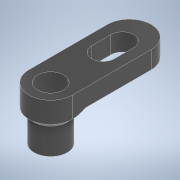
# Autodesk Inventor part: Servo steering actuator
Saved by Autodesk Inventor 2022.6 (Build 266554000, 554)
## iProperties
Created: 2024-11-03
Part Number: Servo steering actuator
Material: Generic
Document SubType Name: Modeling
Designer: Zhong
Density: 1 g/cm^3
Appearance: Dark Gray
Author: Zhong
Autodesk Inventor part; units mm, degrees
ref_plane "YZ Plane" through (0, 0, 0) normal (1, 0, 0) x (0, 1, 0)
ref_plane "XZ Plane" through (0, 0, 0) normal (0, 1, 0) x (-1, 0, 0)
ref_plane "XY Plane" through (0, 0, 0) normal (0, 0, 1) x (1, 0, 0)
sketch "Sketch1" plane through (0, 0, 0) normal (0, 1, 0) x (-1, 0, 0)
  circle A0 centre (0, 0) radius 1.4
  circle A1 centre (0, 0) radius 5
  circle A2 centre (0, -18) radius 5
  line L0 (5, 0) -> (5, -18)
  line L1 (-5, -18) -> (-5, 0)
  dimension "d0" = 2.8
  dimension "d1" = 10
  dimension "d3" = 18
  constraints: 4 end point, 4 point on circle, 4 tangent, 3 centre point, 2 coincident, 1 equal radius, 1 vertical alignment
  measures "d0" diameter of A0
  measures "d1" diameter of A1
  measures "d3" distance of point (0, 0) A2.centre
extrude "Extrusion1" add sketch "Sketch1" along normal blind 4
sketch "Sketch2" plane through (0, 4, 0) normal (0, 1, 0) x (1, 0, 0)
  line L0 (-5, 18) -> (-5, 0) projected
  arc A0 (-5, 0) -> (5, 0) centre (0, 0) ccw projected
  line L1 (5, 0) -> (5, 18) projected
  arc A1 (5, 18) -> (-5, 18) centre (0, 18) ccw projected
  circle A2 centre (0, 0) radius 1.4 projected
  line L2 (0, 16.4) -> (0, 12) construction
  line L3 (-2.6, 16.4) -> (-2.6, 12)
  line L4 (2.6, 12) -> (2.6, 16.4)
  arc A3 (2.6, 16.4) -> (-2.6, 16.4) centre (0, 16.4) ccw
  arc A4 (-2.6, 12) -> (2.6, 12) centre (0, 12) ccw
  point P0 (0, 14.2)
  dimension "d6" = 4.4
  dimension "d7" = 5.2
  dimension "d9" = 12
  constraints: 8 end point, 4 point on circle, 4 tangent, 2 centre point, 1 midpoint, 1 parallel, 1 vertical, 1 vertical alignment
  measures "d6" distance of L2.start L2.end
  measures "d7" diameter of A4
  measures "d9" distance of point (0, 0) L2.end
extrude "Extrusion2" cut sketch "Sketch2" against normal through all contours A3 L4 A4 L3
sketch "Sketch4" plane through (0, 0, 0) normal (0, -1, 0) x (1, 0, 0)
  line L0 (2.6, -12) -> (2.6, -16.4) projected
  arc A0 (-2.6, -16.4) -> (2.6, -16.4) centre (0, -16.4) ccw projected
  line L1 (-2.6, -16.4) -> (-2.6, -12) projected
  arc A1 (2.6, -12) -> (-2.6, -12) centre (0, -12) ccw projected
  line L2 (-5, -18) -> (-5, 0) projected
  arc A2 (-5, -18) -> (5, -18) centre (0, -18) ccw projected
  line L3 (5, 0) -> (5, -18) projected
  arc A3 (5, 0) -> (-5, 0) centre (0, 0) ccw projected
  circle A4 centre (0, 0) radius 1.4 projected
  arc A5 (5, 0) -> (-5, 0) centre (0, 0) ccw projected
  circle A6 centre (0, 0) radius 1.4 projected
  circle A7 centre (0, 0) radius 3.8
  circle A8 centre (0, 0) radius 1.4
  dimension "d39" = 7.6
  constraints: 2 centre point, 2 coincident, 1 concentric
  measures "d39" diameter of A7
extrude "Extrusion4" add sketch "Sketch4" along normal blind 8 contours A7
sketch "Sketch5" plane through (0, -8, 0) normal (0, -1, 0) x (1, 0, 0)
  circle A0 centre (0, 0) radius 1.4 projected
  circle A1 centre (0, 0) radius 2.5
  dimension "d17" = 5
  constraints: 1 centre point, 1 coincident
  measures "d17" diameter of A1
extrude "Extrusion5" cut sketch "Sketch5" against normal blind 5
sketch "Sketch6" plane through (0, 4, 0) normal (0, 1, 0) x (1, 0, 0)
  arc A0 (-5, 0) -> (5, 0) centre (0, 0) ccw projected
  line L0 (2.6, 16.4) -> (2.6, 12) projected
  arc A1 (-2.6, 12) -> (2.6, 12) centre (0, 12) ccw projected
  line L1 (-2.6, 12) -> (-2.6, 16.4) projected
  arc A2 (2.6, 16.4) -> (-2.6, 16.4) centre (0, 16.4) ccw projected
  line L2 (-5, 18) -> (-5, 0) projected
  arc A3 (-5, 0) -> (5, 0) centre (0, 0) ccw projected
  line L3 (5, 0) -> (5, 18) projected
  arc A4 (5, 18) -> (-5, 18) centre (0, 18) ccw projected
  circle A5 centre (0, 0) radius 1.4 projected
  circle A6 centre (0, 0) radius 1.4 projected
  circle A7 centre (0, 0) radius 3
  dimension "d20" = 6
  constraints: 1 centre point, 1 coincident
  measures "d20" diameter of A7
extrude "Extrusion6" cut sketch "Sketch6" against normal blind 5 contours A7
sketch "Sketch7" plane through (0, -8, 0) normal (0, -1, 0) x (1, 0, 0)
  circle A0 centre (0, 0) radius 2.5 projected
  circle A1 centre (0, 0) radius 2.9
  line L0 (1.9156, 2.1773) -> (1.9156, 1.7248)
  line L1 (1.9156, 1.7248) -> (2.3656, 1.6775)
  line L2 (1.4471, 2.1331) -> (1.8954, 2.1949)
  line L3 (1.3389, 2.5724) -> (1.4471, 2.1331)
  line L4 (0.8946, 2.4174) -> (1.315, 2.5847)
  line L5 (0.6843, 2.8181) -> (0.8946, 2.4174)
  line L6 (0.2901, 2.5613) -> (0.6583, 2.8243)
  line L7 (-0.01, 2.9) -> (0.2901, 2.5613)
  line L8 (-0.3313, 2.5563) -> (-0.0368, 2.8998)
  line L9 (-0.7037, 2.8133) -> (-0.3313, 2.5563)
  line L10 (-0.9334, 2.4027) -> (-0.7296, 2.8067)
  line L11 (-1.3565, 2.5632) -> (-0.9334, 2.4027)
  line L12 (-1.4813, 2.1095) -> (-1.3801, 2.5505)
  line L13 (-1.9305, 2.1641) -> (-1.4813, 2.1095)
  line L14 (-1.9431, 1.6937) -> (-1.9504, 2.1461)
  line L15 (-2.3923, 1.6392) -> (-1.9431, 1.6937)
  line L16 (-2.292, 1.1795) -> (-2.4073, 1.617)
  line L17 (-2.7151, 1.019) -> (-2.292, 1.1795)
  line L18 (-2.5077, 0.5967) -> (-2.7244, 0.9939)
  line L19 (-2.88, 0.3397) -> (-2.5077, 0.5967)
  line L20 (-2.5776, -0.0208) -> (-2.8831, 0.313)
  line L21 (-2.8776, -0.3594) -> (-2.5776, -0.0208)
  line L22 (-2.4977, -0.637) -> (-2.8742, -0.386)
  line L23 (-2.708, -1.0377) -> (-2.4977, -0.637)
  line L24 (-2.2727, -1.2163) -> (-2.6983, -1.0626)
  line L25 (-2.381, -1.6556) -> (-2.2727, -1.2163)
  line L26 (-1.9156, -1.7248) -> (-2.3656, -1.6775)
  line L27 (-1.9156, -2.1773) -> (-1.9156, -1.7248)
  line L28 (-1.4471, -2.1331) -> (-1.8954, -2.1949)
  line L29 (-1.3389, -2.5724) -> (-1.4471, -2.1331)
  line L30 (-0.8946, -2.4174) -> (-1.315, -2.5847)
  line L31 (-0.6843, -2.8181) -> (-0.8946, -2.4174)
  line L32 (-0.2901, -2.5613) -> (-0.6583, -2.8243)
  line L33 (0.01, -2.9) -> (-0.2901, -2.5613)
  line L34 (0.3313, -2.5563) -> (0.0368, -2.8998)
  line L35 (0.7037, -2.8133) -> (0.3313, -2.5563)
  line L36 (0.9334, -2.4027) -> (0.7296, -2.8067)
  line L37 (1.3565, -2.5632) -> (0.9334, -2.4027)
  line L38 (1.4813, -2.1095) -> (1.3801, -2.5505)
  line L39 (1.9305, -2.1641) -> (1.4813, -2.1095)
  line L40 (1.9431, -1.6937) -> (1.9504, -2.1461)
  line L41 (2.3923, -1.6392) -> (1.9431, -1.6937)
  line L42 (2.292, -1.1795) -> (2.4073, -1.617)
  line L43 (2.7151, -1.019) -> (2.292, -1.1795)
  line L44 (2.5077, -0.5967) -> (2.7244, -0.9939)
  line L45 (2.88, -0.3397) -> (2.5077, -0.5967)
  line L46 (2.5776, 0.0208) -> (2.8831, -0.313)
  line L47 (2.8776, 0.3594) -> (2.5776, 0.0208)
  line L48 (2.4977, 0.637) -> (2.8742, 0.386)
  line L49 (2.708, 1.0377) -> (2.4977, 0.637)
  line L50 (2.2727, 1.2163) -> (2.6983, 1.0626)
  line L51 (2.381, 1.6556) -> (2.2727, 1.2163)
  point P0 (2.381, 1.6556)
  point P1 (1.8954, 2.1949)
  point P2 (1.3389, 2.5724)
  point P3 (1.315, 2.5847)
  point P4 (0.6843, 2.8181)
  point P5 (0.6583, 2.8243)
  point P6 (-0.01, 2.9)
  point P7 (-0.0368, 2.8998)
  point P8 (-0.7037, 2.8133)
  point P9 (-0.7296, 2.8067)
  point P10 (-1.3565, 2.5632)
  point P11 (-1.3801, 2.5505)
  point P12 (-1.9305, 2.1641)
  point P13 (-1.9504, 2.1461)
  point P14 (-2.3923, 1.6392)
  point P15 (-2.4073, 1.617)
  point P16 (-2.7151, 1.019)
  point P17 (-2.7244, 0.9939)
  point P18 (-2.88, 0.3397)
  point P19 (-2.8831, 0.313)
  point P20 (-2.8776, -0.3594)
  point P21 (-2.8742, -0.386)
  point P22 (-2.708, -1.0377)
  point P23 (-2.6983, -1.0626)
  point P24 (-2.381, -1.6556)
  point P25 (-2.3656, -1.6775)
  point P26 (-1.9156, -2.1773)
  point P27 (-1.8954, -2.1949)
  point P28 (-1.3389, -2.5724)
  point P29 (-1.315, -2.5847)
  point P30 (-0.6843, -2.8181)
  point P31 (-0.6583, -2.8243)
  point P32 (0.01, -2.9)
  point P33 (0.0368, -2.8998)
  point P34 (0.7037, -2.8133)
  point P35 (0.7296, -2.8067)
  point P36 (1.3565, -2.5632)
  point P37 (1.3801, -2.5505)
  point P38 (1.9305, -2.1641)
  point P39 (1.9504, -2.1461)
  point P40 (2.3923, -1.6392)
  point P41 (2.4073, -1.617)
  point P42 (2.7151, -1.019)
  point P43 (2.7244, -0.9939)
  point P44 (2.88, -0.3397)
  point P45 (2.8831, -0.313)
  point P46 (2.8776, 0.3594)
  point P47 (2.8742, 0.386)
  point P48 (2.708, 1.0377)
  point P49 (2.6983, 1.0626)
  dimension "d24" = 5.8
  dimension "d30" = 96
  dimension "d31" = 0.45
  dimension "d34" = 360
  constraints: 104 end point, 1 coincident, 1 equal length, 1 vertical, 135 other
  measures "d30" angle of L0 L1
  measures "d31" horizontal distance of L0.end L1.end
extrude "Extrusion7" cut sketch "Sketch7" against normal up to surface (5 mm away) contours L47 L46 A1 L45 L44 L43 L42 L41 L40 L39 L38 L37 L36 L35 L34 L33 L32 L31 L30 L29 L28 L27 L26 L25 L24 L23 L22 L21 L20 L19 L18 L17 L16 L15 L14 L13 L12 L11 L10 L9 L8 L7 L6 L5 L4 L3 L2 L0 L1 L51 L50 L49 L48
chamfer "Chamfer1" distance 2 angle 45 1 edges at (-3.8, 0, 0)
body "Solid1"
